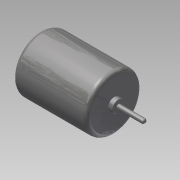
# Autodesk Inventor part: Kipas
Saved by Autodesk Inventor 2015 SP1 (Build 190203100, 203)
## iProperties
Created: 2015-02-02
Part Number: Kipas
Material: Generic
Document SubType Name: Modeling
Designer: Rafi Kurnia Putra
Density: 1 g/cm^3
Appearance: Stainless - Brushed
Mass: 17.089 g
Surface Area: 44.1561 cm^2
Volume: 17.089 cm^3
Author: Rafi Kurnia Putra
Autodesk Inventor part; units mm, degrees
ref_plane "YZ Plane" through (0, 0, 0) normal (1, 0, 0) x (0, 1, 0)
ref_plane "XZ Plane" through (0, 0, 0) normal (0, 1, 0) x (-1, 0, 0)
ref_plane "XY Plane" through (0, 0, 0) normal (0, 0, 1) x (1, 0, 0)
sketch "Sketch1" plane through (0, 0, 0) normal (0, 0, 1) x (1, 0, 0)
  circle A0 centre (0, 0) radius 12.685
  circle A1 centre (0, 0) radius 2.83
  circle A2 centre (0, 0) radius 1.05
  dimension "d0" = 25.37
  dimension "d1" = 5.66
  dimension "d2" = 2.1
  constraints: 3 centre point, 3 coincident
  measures "d0" diameter of A0
  measures "d1" diameter of A1
  measures "d2" diameter of A2
extrude "Extrusion1" add sketch "Sketch1" along normal blind 33.86 contours A0 | A1 | A2
extrude "Extrusion2" add sketch "Sketch1" against normal blind 2 contours A1
extrude "Extrusion3" add sketch "Sketch1" against normal blind 14.28 contours A2
fillet "Fillet1" radius 2 2 edges at (-12.685, 0, 0) (-12.685, 0, 33.86)
fillet "Fillet2" radius 0.25 1 edges at (-2.83, 0, -2)
fillet "Fillet3" radius 1 1 edges at (-1.05, 0, -14.28)
sketch "Sketch2" plane through (0, 0, 33.86) normal (0, 0, 1) x (1, 0, 0)
  circle A0 centre (0, 0) radius 1.05 projected
  circle A1 centre (0, 0) radius 1
  circle A2 centre (0, 0) radius 2.83
  dimension "d12" = 2
  constraints: 2 centre point, 2 coincident
  measures "d12" diameter of A1
extrude "Extrusion4" add sketch "Sketch2" along normal blind 2 contours A2
extrude "Extrusion5" add sketch "Sketch2" along normal blind 2.62 contours A1
fillet "Fillet4" radius 0.25 1 edges at (-2.83, 0, 35.86)
fillet "Fillet5" radius 1 1 edges at (-1, 0, 36.48)
sketch "Sketch4" plane through (0, 0, 33.86) normal (0, 0, 1) x (1, 0, 0)
  circle A0 centre (0, 0) radius 2.83 projected
  circle A1 centre (0, 0) radius 3.6056
  line L0 (-4.1941, 0.5305) -> (-4.1946, 0.524)
  spline S0 degree 2 poles (-4.1946, 0.524) (-4.1996, 0.5098) (-4.2034, 0.4784) (-4.2049, 0.4565) knots 0 0 0 1 2 2 2
  spline S1 degree 2 poles (-4.2049, 0.4565) (-4.2084, 0.4056) (-4.1708, 0.3023) (-4.1303, 0.254) knots 0 0 0 1 2 2 2
  line L1 (-4.1303, 0.254) -> (-3.5991, 0.2175)
  line L2 (-3.5991, 0.2175) -> (-3.6078, 0.0914)
  line L3 (-3.6078, 0.0914) -> (-4.3564, 0.1428)
  line L4 (-4.3564, 0.1428) -> (-4.3477, 0.269)
  line L5 (-4.3477, 0.269) -> (-4.2362, 0.2613)
  spline S2 degree 2 poles (-4.2362, 0.2613) (-4.2929, 0.3342) (-4.336, 0.4404) (-4.3326, 0.4889) knots 0 0 0 1 2 2 2
  spline S3 degree 2 poles (-4.3326, 0.4889) (-4.3313, 0.5083) (-4.3283, 0.5276) (-4.3251, 0.5395) knots 0 0 0 1 2 2 2
  line L6 (-4.3251, 0.5395) -> (-4.1941, 0.5305)
  spline S4 degree 2 poles (-3.5469, 1.0102) (-3.5395, 0.9926) (-3.5123, 0.9326) (-3.5062, 0.9061) knots 0 0 0 1 2 2 2
  spline S5 degree 2 poles (-3.5062, 0.9061) (-3.4967, 0.8697) (-3.4932, 0.8046) (-3.5065, 0.7495) knots 0 0 0 1 2 2 2
  spline S6 degree 2 poles (-3.5065, 0.7495) (-3.5174, 0.7046) (-3.5709, 0.6317) (-3.609, 0.6084) knots 0 0 0 1 2 2 2
  spline S7 degree 2 poles (-3.609, 0.6084) (-3.646, 0.5864) (-3.7428, 0.5723) (-3.7916, 0.5841) knots 0 0 0 1 2 2 2
  spline S8 degree 2 poles (-3.7916, 0.5841) (-3.8672, 0.6024) (-3.9589, 0.6921) (-3.9729, 0.7688) knots 0 0 0 1 2 2 2
  spline S9 degree 2 poles (-3.9729, 0.7688) (-3.9864, 0.8371) (-3.9673, 1.0093) (-3.9494, 1.1075) knots 0 0 0 1 2 2 2
  line L7 (-3.9494, 1.1075) -> (-3.9731, 1.1132)
  spline S10 degree 2 poles (-3.9731, 1.1132) (-4.0156, 1.1235) (-4.0747, 1.1102) (-4.0953, 1.0902) knots 0 0 0 1 2 2 2
  spline S11 degree 2 poles (-4.0953, 1.0902) (-4.116, 1.0702) (-4.1418, 1.0047) (-4.1506, 0.9685) knots 0 0 0 1 2 2 2
  spline S12 degree 2 poles (-4.1506, 0.9685) (-4.1609, 0.926) (-4.1635, 0.8049) (-4.1529, 0.7415) knots 0 0 0 1 2 2 2
  line L8 (-4.1529, 0.7415) -> (-4.1546, 0.7344)
  line L9 (-4.1546, 0.7344) -> (-4.2799, 0.7647)
  spline S13 degree 2 poles (-4.2799, 0.7647) (-4.2812, 0.8008) (-4.2741, 0.9333) (-4.2591, 0.9956) knots 0 0 0 1 2 2 2
  spline S14 degree 2 poles (-4.2591, 0.9956) (-4.2408, 1.0712) (-4.1923, 1.1687) (-4.1516, 1.2022) knots 0 0 0 1 2 2 2
  spline S15 degree 2 poles (-4.1516, 1.2022) (-4.112, 1.2351) (-4.0072, 1.2515) (-3.9386, 1.2349) knots 0 0 0 1 2 2 2
  line L10 (-3.9386, 1.2349) -> (-3.44, 1.1144)
  line L11 (-3.44, 1.1144) -> (-3.4697, 0.9915)
  line L12 (-3.4697, 0.9915) -> (-3.5469, 1.0102)
  line L13 (-3.6493, 1.0349) -> (-3.8518, 1.0839)
  spline S16 degree 2 poles (-3.8518, 1.0839) (-3.8585, 1.0388) (-3.8773, 0.9025) (-3.8747, 0.8577) knots 0 0 0 1 2 2 2
  spline S17 degree 2 poles (-3.8747, 0.8577) (-3.8716, 0.8052) (-3.8248, 0.7264) (-3.7696, 0.713) knots 0 0 0 1 2 2 2
  spline S18 degree 2 poles (-3.7696, 0.713) (-3.7066, 0.6978) (-3.6257, 0.7533) (-3.6093, 0.821) knots 0 0 0 1 2 2 2
  spline S19 degree 2 poles (-3.6093, 0.821) (-3.5954, 0.8785) (-3.6222, 0.985) (-3.6493, 1.0349) knots 0 0 0 1 2 2 2
  line L14 (-4.0695, 2.0028) -> (-4.072, 1.9968)
  spline S20 degree 2 poles (-4.072, 1.9968) (-4.0846, 1.9837) (-4.1198, 1.9299) (-4.1296, 1.9068) knots 0 0 0 1 2 2 2
  spline S21 degree 2 poles (-4.1296, 1.9068) (-4.1607, 1.8337) (-4.1216, 1.7432) (-4.0351, 1.7064) knots 0 0 0 1 2 2 2
  line L15 (-4.0351, 1.7064) -> (-4.012, 1.6966)
  line L16 (-4.012, 1.6966) -> (-3.9303, 1.8891)
  line L17 (-3.9303, 1.8891) -> (-3.834, 1.8482)
  line L18 (-3.834, 1.8482) -> (-3.9142, 1.6595)
  line L19 (-3.9142, 1.6595) -> (-3.3197, 1.407)
  line L20 (-3.3197, 1.407) -> (-3.3691, 1.2907)
  line L21 (-3.3691, 1.2907) -> (-3.9636, 1.5431)
  line L22 (-3.9636, 1.5431) -> (-3.9968, 1.4648)
  line L23 (-3.9968, 1.4648) -> (-4.0931, 1.5057)
  line L24 (-4.0931, 1.5057) -> (-4.0598, 1.584)
  line L25 (-4.0598, 1.584) -> (-4.0829, 1.5938)
  spline S22 degree 2 poles (-4.0829, 1.5938) (-4.2067, 1.6464) (-4.2855, 1.8216) (-4.238, 1.9335) knots 0 0 0 1 2 2 2
  spline S23 degree 2 poles (-4.238, 1.9335) (-4.2244, 1.9655) (-4.1914, 2.0246) (-4.1762, 2.0481) knots 0 0 0 1 2 2 2
  line L26 (-4.1762, 2.0481) -> (-4.0695, 2.0028)
  line L27 (-3.1163, 1.8146) -> (-3.178, 1.7043)
  line L28 (-3.178, 1.7043) -> (-3.8329, 2.0705)
  line L29 (-3.8329, 2.0705) -> (-3.7713, 2.1808)
  line L30 (-3.7713, 2.1808) -> (-3.1163, 1.8146)
  line L31 (-3.8758, 2.2495) -> (-3.9458, 2.1243)
  line L32 (-3.9458, 2.1243) -> (-4.0604, 2.1884)
  line L33 (-4.0604, 2.1884) -> (-3.9904, 2.3136)
  line L34 (-3.9904, 2.3136) -> (-3.8758, 2.2495)
  line L35 (-2.6508, 2.472) -> (-2.7511, 2.3395)
  line L36 (-2.7511, 2.3395) -> (-3.2082, 2.3359)
  line L37 (-3.2082, 2.3359) -> (-3.1997, 2.2665)
  line L38 (-3.1997, 2.2665) -> (-2.9497, 2.0772)
  line L39 (-2.9497, 2.0772) -> (-3.026, 1.9764)
  line L40 (-3.026, 1.9764) -> (-3.8588, 2.6069)
  line L41 (-3.8588, 2.6069) -> (-3.7825, 2.7077)
  line L42 (-3.7825, 2.7077) -> (-3.2953, 2.3389)
  line L43 (-3.2953, 2.3389) -> (-3.3689, 2.7666)
  line L44 (-3.3689, 2.7666) -> (-3.274, 2.892)
  line L45 (-3.274, 2.892) -> (-3.2099, 2.4572)
  line L46 (-3.2099, 2.4572) -> (-2.6508, 2.472)
  line L47 (-2.1644, 2.8983) -> (-2.2593, 2.8148)
  line L48 (-2.2593, 2.8148) -> (-2.3139, 2.8768)
  spline S24 degree 2 poles (-2.3139, 2.8768) (-2.324, 2.7999) (-2.3676, 2.6913) (-2.4162, 2.6484) knots 0 0 0 1 2 2 2
  spline S25 degree 2 poles (-2.4162, 2.6484) (-2.4527, 2.6163) (-2.5392, 2.5833) (-2.586, 2.5886) knots 0 0 0 1 2 2 2
  spline S26 degree 2 poles (-2.586, 2.5886) (-2.6333, 2.5933) (-2.7302, 2.6494) (-2.7806, 2.7065) knots 0 0 0 1 2 2 2
  line L49 (-2.7806, 2.7065) -> (-3.1025, 3.072)
  line L50 (-3.1025, 3.072) -> (-3.0077, 3.1556)
  line L51 (-3.0077, 3.1556) -> (-2.7248, 2.8345)
  spline S27 degree 2 poles (-2.7248, 2.8345) (-2.6852, 2.7895) (-2.6265, 2.7364) (-2.5957, 2.7247) knots 0 0 0 1 2 2 2
  spline S28 degree 2 poles (-2.5957, 2.7247) (-2.5649, 2.713) (-2.5077, 2.7277) (-2.4706, 2.7604) knots 0 0 0 1 2 2 2
  spline S29 degree 2 poles (-2.4706, 2.7604) (-2.4359, 2.7909) (-2.3923, 2.8996) (-2.3846, 2.9571) knots 0 0 0 1 2 2 2
  line L52 (-2.3846, 2.9571) -> (-2.7553, 3.3779)
  line L53 (-2.7553, 3.3779) -> (-2.6605, 3.4614)
  line L54 (-2.6605, 3.4614) -> (-2.1644, 2.8983)
  line L55 (-1.9912, 3.7292) -> (-1.9968, 3.7258)
  spline S30 degree 2 poles (-1.9968, 3.7258) (-2.0113, 3.7217) (-2.0391, 3.7066) (-2.0578, 3.6952) knots 0 0 0 1 2 2 2
  spline S31 degree 2 poles (-2.0578, 3.6952) (-2.1014, 3.6687) (-2.164, 3.5783) (-2.18, 3.5173) knots 0 0 0 1 2 2 2
  line L56 (-2.18, 3.5173) -> (-1.9028, 3.0627)
  line L57 (-1.9028, 3.0627) -> (-2.0107, 2.9969)
  line L58 (-2.0107, 2.9969) -> (-2.4014, 3.6376)
  line L59 (-2.4014, 3.6376) -> (-2.2935, 3.7034)
  line L60 (-2.2935, 3.7034) -> (-2.2352, 3.6079)
  spline S32 degree 2 poles (-2.2352, 3.6079) (-2.2085, 3.6964) (-2.1468, 3.7929) (-2.1053, 3.8182) knots 0 0 0 1 2 2 2
  spline S33 degree 2 poles (-2.1053, 3.8182) (-2.0887, 3.8283) (-2.0712, 3.837) (-2.0596, 3.8413) knots 0 0 0 1 2 2 2
  line L61 (-2.0596, 3.8413) -> (-1.9912, 3.7292)
  line L62 (-1.037, 3.466) -> (-1.1547, 3.4199)
  line L63 (-1.1547, 3.4199) -> (-1.3106, 3.8184)
  spline S34 degree 2 poles (-1.3106, 3.8184) (-1.3295, 3.8667) (-1.3711, 3.9461) (-1.3944, 3.9657) knots 0 0 0 1 2 2 2
  spline S35 degree 2 poles (-1.3944, 3.9657) (-1.4191, 3.9865) (-1.4805, 3.9921) (-1.5242, 3.975) knots 0 0 0 1 2 2 2
  spline S36 degree 2 poles (-1.5242, 3.975) (-1.568, 3.9578) (-1.6425, 3.8747) (-1.6723, 3.8196) knots 0 0 0 1 2 2 2
  line L64 (-1.6723, 3.8196) -> (-1.4679, 3.2974)
  line L65 (-1.4679, 3.2974) -> (-1.5856, 3.2513)
  line L66 (-1.5856, 3.2513) -> (-1.8591, 3.9501)
  line L67 (-1.8591, 3.9501) -> (-1.7414, 3.9962)
  line L68 (-1.7414, 3.9962) -> (-1.7109, 3.9184)
  spline S37 degree 2 poles (-1.7109, 3.9184) (-1.6767, 3.9867) (-1.5943, 4.0763) (-1.537, 4.0988) knots 0 0 0 1 2 2 2
  spline S38 degree 2 poles (-1.537, 4.0988) (-1.4344, 4.1389) (-1.265, 4.0486) (-1.2145, 3.9195) knots 0 0 0 1 2 2 2
  line L69 (-1.2145, 3.9195) -> (-1.037, 3.466)
  line L70 (-0.7376, 3.5299) -> (-0.8609, 3.5018)
  line L71 (-0.8609, 3.5018) -> (-1.0272, 4.2336)
  line L72 (-1.0272, 4.2336) -> (-0.9039, 4.2616)
  line L73 (-0.9039, 4.2616) -> (-0.7376, 3.5299)
  line L74 (-0.9229, 4.3853) -> (-1.0628, 4.3535)
  line L75 (-1.0628, 4.3535) -> (-1.0919, 4.4815)
  line L76 (-1.0919, 4.4815) -> (-0.952, 4.5133)
  line L77 (-0.952, 4.5133) -> (-0.9229, 4.3853)
  spline S39 degree 2 poles (-0.1468, 3.685) (-0.1613, 3.6725) (-0.2097, 3.628) (-0.233, 3.6139) knots 0 0 0 1 2 2 2
  spline S40 degree 2 poles (-0.233, 3.6139) (-0.2647, 3.5935) (-0.3254, 3.5699) (-0.3819, 3.5653) knots 0 0 0 1 2 2 2
  spline S41 degree 2 poles (-0.3819, 3.5653) (-0.428, 3.5617) (-0.514, 3.5897) (-0.548, 3.6187) knots 0 0 0 1 2 2 2
  spline S42 degree 2 poles (-0.548, 3.6187) (-0.5803, 3.647) (-0.624, 3.7345) (-0.628, 3.7846) knots 0 0 0 1 2 2 2
  spline S43 degree 2 poles (-0.628, 3.7846) (-0.6342, 3.8621) (-0.5776, 3.9773) (-0.5091, 4.0145) knots 0 0 0 1 2 2 2
  spline S44 degree 2 poles (-0.5091, 4.0145) (-0.4484, 4.0486) (-0.2789, 4.0842) (-0.18, 4.0978) knots 0 0 0 1 2 2 2
  line L78 (-0.18, 4.0978) -> (-0.1819, 4.122)
  spline S45 degree 2 poles (-0.1819, 4.122) (-0.1854, 4.1657) (-0.2164, 4.2176) (-0.2419, 4.231) knots 0 0 0 1 2 2 2
  spline S46 degree 2 poles (-0.2419, 4.231) (-0.2674, 4.2444) (-0.3376, 4.2486) (-0.3748, 4.2456) knots 0 0 0 1 2 2 2
  spline S47 degree 2 poles (-0.3748, 4.2456) (-0.4184, 4.2421) (-0.5343, 4.2068) (-0.5912, 4.177) knots 0 0 0 1 2 2 2
  line L79 (-0.5912, 4.177) -> (-0.5985, 4.1764)
  line L80 (-0.5985, 4.1764) -> (-0.6088, 4.3048)
  spline S48 degree 2 poles (-0.6088, 4.3048) (-0.5748, 4.3173) (-0.4467, 4.352) (-0.3829, 4.3571) knots 0 0 0 1 2 2 2
  spline S49 degree 2 poles (-0.3829, 4.3571) (-0.3054, 4.3633) (-0.1976, 4.3476) (-0.1531, 4.3195) knots 0 0 0 1 2 2 2
  spline S50 degree 2 poles (-0.1531, 4.3195) (-0.1094, 4.2921) (-0.0612, 4.1976) (-0.0555, 4.1273) knots 0 0 0 1 2 2 2
  line L81 (-0.0555, 4.1273) -> (-0.0145, 3.616)
  line L82 (-0.0145, 3.616) -> (-0.1405, 3.6059)
  line L83 (-0.1405, 3.6059) -> (-0.1468, 3.685)
  line L84 (-0.1553, 3.7901) -> (-0.1719, 3.9977)
  spline S51 degree 2 poles (-0.1719, 3.9977) (-0.2168, 3.99) (-0.3523, 3.9653) (-0.394, 3.9489) knots 0 0 0 1 2 2 2
  spline S52 degree 2 poles (-0.394, 3.9489) (-0.4429, 3.9295) (-0.5032, 3.8605) (-0.4986, 3.8039) knots 0 0 0 1 2 2 2
  spline S53 degree 2 poles (-0.4986, 3.8039) (-0.4935, 3.7393) (-0.4155, 3.6797) (-0.346, 3.6853) knots 0 0 0 1 2 2 2
  spline S54 degree 2 poles (-0.346, 3.6853) (-0.2871, 3.69) (-0.1942, 3.7487) (-0.1553, 3.7901) knots 0 0 0 1 2 2 2
  point P0 (0, 3.6056)
  point P1 (-3.6056, 0)
  constraints: 2 point on circle, 1 centre point, 1 other
extrude "Extrusion6" cut sketch "Sketch4" against normal blind 10 contours L2 L3 L4 L5 S2 S3 L6 L0 S0 S1 L1 | L20 L21 L22 L23 L24 L25 S22 S23 L26 L14 S20 S21 L15 L16 L17 L18 L19 | L57 L58 L59 L60 S32 S33 L61 L55 S30 S31 L56 | A1 L71 L72 L73 | S41 S42 S43 S44 L78 S45 S46 S47 L79 L80 S48 S49 S50 L81 L82 L83 S39 S40 A1 | A1 S40 S41 | S24 S25 A1 | A1 S25 S26 L49 L50 L51 S27 S28 S29 L52 L53 L54 L47 L48 S24 | A1 L28 L29 L30 | S6 S7 S8 S9 L7 S10 S11 S12 L8 L9 S13 S14 S15 L10 L11 L12 S4 S5 A1 | A1 S5 S6 | L31 L32 L33 L34 | L35 L36 L37 L38 L39 L40 L41 L42 L43 L44 L45 L46 | L62 L63 S34 S35 S36 L64 L65 L66 L67 L68 S37 S38 L69 | L74 L75 L76 L77
sketch "Sketch5" plane through (0, 0, 0) normal (0, 0, -1) x (-1, 0, 0)
  circle A0 centre (0, 0) radius 10.685 projected
  line L0 (-4.7473, -8.884) -> (-4.7529, -8.8808)
  spline S0 degree 2 poles (-4.7529, -8.8808) (-4.7636, -8.8701) (-4.7903, -8.8531) (-4.8094, -8.8424) knots 0 0 0 1 2 2 2
  spline S1 degree 2 poles (-4.8094, -8.8424) (-4.8538, -8.8172) (-4.9632, -8.8065) (-5.0242, -8.8223) knots 0 0 0 1 2 2 2
  line L1 (-5.0242, -8.8223) -> (-5.2864, -9.2857)
  line L2 (-5.2864, -9.2857) -> (-5.3964, -9.2235)
  line L3 (-5.3964, -9.2235) -> (-5.027, -8.5703)
  line L4 (-5.027, -8.5703) -> (-4.9169, -8.6325)
  line L5 (-4.9169, -8.6325) -> (-4.972, -8.7299)
  spline S2 degree 2 poles (-4.972, -8.7299) (-4.8817, -8.7102) (-4.7674, -8.7171) (-4.7251, -8.7411) knots 0 0 0 1 2 2 2
  spline S3 degree 2 poles (-4.7251, -8.7411) (-4.7081, -8.7506) (-4.692, -8.7616) (-4.6826, -8.7697) knots 0 0 0 1 2 2 2
  line L6 (-4.6826, -8.7697) -> (-4.7473, -8.884)
  spline S4 degree 2 poles (-4.5536, -9.5794) (-4.5724, -9.5828) (-4.6368, -9.5962) (-4.664, -9.5964) knots 0 0 0 1 2 2 2
  spline S5 degree 2 poles (-4.664, -9.5964) (-4.7017, -9.5977) (-4.7659, -9.5868) (-4.8168, -9.5618) knots 0 0 0 1 2 2 2
  spline S6 degree 2 poles (-4.8168, -9.5618) (-4.8582, -9.5414) (-4.9177, -9.4732) (-4.9321, -9.4309) knots 0 0 0 1 2 2 2
  spline S7 degree 2 poles (-4.9321, -9.4309) (-4.9454, -9.39) (-4.938, -9.2925) (-4.9158, -9.2474) knots 0 0 0 1 2 2 2
  spline S8 degree 2 poles (-4.9158, -9.2474) (-4.8814, -9.1776) (-4.7738, -9.1078) (-4.6959, -9.1109) knots 0 0 0 1 2 2 2
  spline S9 degree 2 poles (-4.6959, -9.1109) (-4.6263, -9.1127) (-4.4625, -9.169) (-4.3706, -9.208) knots 0 0 0 1 2 2 2
  line L7 (-4.3706, -9.208) -> (-4.3598, -9.1861)
  spline S10 degree 2 poles (-4.3598, -9.1861) (-4.3405, -9.1469) (-4.3405, -9.0864) (-4.3555, -9.0618) knots 0 0 0 1 2 2 2
  spline S11 degree 2 poles (-4.3555, -9.0618) (-4.3705, -9.0373) (-4.4287, -8.9977) (-4.4622, -8.9813) knots 0 0 0 1 2 2 2
  spline S12 degree 2 poles (-4.4622, -8.9813) (-4.5014, -8.9619) (-4.619, -8.9329) (-4.6832, -8.9293) knots 0 0 0 1 2 2 2
  line L8 (-4.6832, -8.9293) -> (-4.6897, -8.9261)
  line L9 (-4.6897, -8.9261) -> (-4.6328, -8.8105)
  spline S13 degree 2 poles (-4.6328, -8.8105) (-4.5972, -8.8172) (-4.4694, -8.853) (-4.412, -8.8813) knots 0 0 0 1 2 2 2
  spline S14 degree 2 poles (-4.412, -8.8813) (-4.3422, -8.9157) (-4.2577, -8.9844) (-4.2339, -9.0314) knots 0 0 0 1 2 2 2
  spline S15 degree 2 poles (-4.2339, -9.0314) (-4.2104, -9.0773) (-4.2174, -9.1831) (-4.2486, -9.2464) knots 0 0 0 1 2 2 2
  line L10 (-4.2486, -9.2464) -> (-4.4753, -9.7065)
  line L11 (-4.4753, -9.7065) -> (-4.5887, -9.6507)
  line L12 (-4.5887, -9.6507) -> (-4.5536, -9.5794)
  line L13 (-4.507, -9.4849) -> (-4.415, -9.2981)
  spline S16 degree 2 poles (-4.415, -9.2981) (-4.4575, -9.2817) (-4.5864, -9.2335) (-4.6307, -9.2262) knots 0 0 0 1 2 2 2
  spline S17 degree 2 poles (-4.6307, -9.2262) (-4.6826, -9.2178) (-4.7697, -9.2462) (-4.7948, -9.2971) knots 0 0 0 1 2 2 2
  spline S18 degree 2 poles (-4.7948, -9.2971) (-4.8235, -9.3552) (-4.787, -9.4463) (-4.7245, -9.4771) knots 0 0 0 1 2 2 2
  spline S19 degree 2 poles (-4.7245, -9.4771) (-4.6715, -9.5033) (-4.5617, -9.5005) (-4.507, -9.4849) knots 0 0 0 1 2 2 2
  line L14 (-3.5881, -9.0822) -> (-3.594, -9.0796)
  spline S20 degree 2 poles (-3.594, -9.0796) (-3.6072, -9.067) (-3.6609, -9.0318) (-3.684, -9.022) knots 0 0 0 1 2 2 2
  spline S21 degree 2 poles (-3.684, -9.022) (-3.7571, -8.9909) (-3.8476, -9.0299) (-3.8844, -9.1164) knots 0 0 0 1 2 2 2
  line L15 (-3.8844, -9.1164) -> (-3.8943, -9.1395)
  line L16 (-3.8943, -9.1395) -> (-3.7019, -9.2214)
  line L17 (-3.7019, -9.2214) -> (-3.7428, -9.3176)
  line L18 (-3.7428, -9.3176) -> (-3.9315, -9.2373)
  line L19 (-3.9315, -9.2373) -> (-4.1842, -9.8317)
  line L20 (-4.1842, -9.8317) -> (-4.3006, -9.7822)
  line L21 (-4.3006, -9.7822) -> (-4.0478, -9.1878)
  line L22 (-4.0478, -9.1878) -> (-4.1261, -9.1545)
  line L23 (-4.1261, -9.1545) -> (-4.0852, -9.0583)
  line L24 (-4.0852, -9.0583) -> (-4.0069, -9.0916)
  line L25 (-4.0069, -9.0916) -> (-3.997, -9.0685)
  spline S22 degree 2 poles (-3.997, -9.0685) (-3.9444, -8.9447) (-3.7691, -8.866) (-3.6573, -8.9136) knots 0 0 0 1 2 2 2
  spline S23 degree 2 poles (-3.6573, -8.9136) (-3.6252, -8.9272) (-3.5662, -8.9603) (-3.5427, -8.9755) knots 0 0 0 1 2 2 2
  line L26 (-3.5427, -8.9755) -> (-3.5881, -9.0822)
  line L27 (-3.7609, -10.0015) -> (-3.8789, -9.9563)
  line L28 (-3.8789, -9.9563) -> (-3.6107, -9.2555)
  line L29 (-3.6107, -9.2555) -> (-3.4926, -9.3006)
  line L30 (-3.4926, -9.3006) -> (-3.7609, -10.0015)
  line L31 (-3.4396, -9.1873) -> (-3.5736, -9.136)
  line L32 (-3.5736, -9.136) -> (-3.5267, -9.0134)
  line L33 (-3.5267, -9.0134) -> (-3.3927, -9.0647)
  line L34 (-3.3927, -9.0647) -> (-3.4396, -9.1873)
  line L35 (-2.9974, -10.2627) -> (-3.1551, -10.2106)
  line L36 (-3.1551, -10.2106) -> (-3.3063, -9.7792)
  line L37 (-3.3063, -9.7792) -> (-3.3692, -9.8097)
  line L38 (-3.3692, -9.8097) -> (-3.4676, -10.1075)
  line L39 (-3.4676, -10.1075) -> (-3.5876, -10.0678)
  line L40 (-3.5876, -10.0678) -> (-3.2602, -9.0759)
  line L41 (-3.2602, -9.0759) -> (-3.1401, -9.1155)
  line L42 (-3.1401, -9.1155) -> (-3.3316, -9.6958)
  line L43 (-3.3316, -9.6958) -> (-2.9507, -9.4879)
  line L44 (-2.9507, -9.4879) -> (-2.8014, -9.5371)
  line L45 (-2.8014, -9.5371) -> (-3.1921, -9.7384)
  line L46 (-3.1921, -9.7384) -> (-2.9974, -10.2627)
  line L47 (-2.3708, -10.4227) -> (-2.4933, -10.3914)
  line L48 (-2.4933, -10.3914) -> (-2.4727, -10.3113)
  spline S24 degree 2 poles (-2.4727, -10.3113) (-2.5419, -10.3462) (-2.6563, -10.3713) (-2.7191, -10.3552) knots 0 0 0 1 2 2 2
  spline S25 degree 2 poles (-2.7191, -10.3552) (-2.7662, -10.3431) (-2.8421, -10.2902) (-2.8641, -10.2486) knots 0 0 0 1 2 2 2
  spline S26 degree 2 poles (-2.8641, -10.2486) (-2.8868, -10.2068) (-2.895, -10.0951) (-2.8761, -10.0213) knots 0 0 0 1 2 2 2
  line L49 (-2.8761, -10.0213) -> (-2.7551, -9.5495)
  line L50 (-2.7551, -9.5495) -> (-2.6327, -9.5809)
  line L51 (-2.6327, -9.5809) -> (-2.7389, -9.9954)
  spline S27 degree 2 poles (-2.7389, -9.9954) (-2.7538, -10.0535) (-2.7647, -10.1319) (-2.757, -10.1639) knots 0 0 0 1 2 2 2
  spline S28 degree 2 poles (-2.757, -10.1639) (-2.7494, -10.196) (-2.705, -10.235) (-2.6571, -10.2473) knots 0 0 0 1 2 2 2
  spline S29 degree 2 poles (-2.6571, -10.2473) (-2.6124, -10.2588) (-2.498, -10.2337) (-2.4462, -10.2077) knots 0 0 0 1 2 2 2
  line L52 (-2.4462, -10.2077) -> (-2.3069, -9.6645)
  line L53 (-2.3069, -9.6645) -> (-2.1845, -9.6958)
  line L54 (-2.1845, -9.6958) -> (-2.3708, -10.4227)
  line L55 (-1.6835, -9.9311) -> (-1.6898, -9.9299)
  spline S30 degree 2 poles (-1.6898, -9.9299) (-1.7034, -9.9232) (-1.7341, -9.9155) (-1.7556, -9.9114) knots 0 0 0 1 2 2 2
  spline S31 degree 2 poles (-1.7556, -9.9114) (-1.8057, -9.9016) (-1.9128, -9.9262) (-1.9657, -9.9605) knots 0 0 0 1 2 2 2
  line L56 (-1.9657, -9.9605) -> (-2.0673, -10.4832)
  line L57 (-2.0673, -10.4832) -> (-2.1914, -10.459)
  line L58 (-2.1914, -10.459) -> (-2.0482, -9.7224)
  line L59 (-2.0482, -9.7224) -> (-1.9241, -9.7465)
  line L60 (-1.9241, -9.7465) -> (-1.9455, -9.8563)
  spline S32 degree 2 poles (-1.9455, -9.8563) (-1.8661, -9.809) (-1.7555, -9.7793) (-1.7078, -9.7886) knots 0 0 0 1 2 2 2
  spline S33 degree 2 poles (-1.7078, -9.7886) (-1.6887, -9.7923) (-1.6699, -9.7976) (-1.6584, -9.8023) knots 0 0 0 1 2 2 2
  line L61 (-1.6584, -9.8023) -> (-1.6835, -9.9311)
  line L62 (-1.1204, -10.6303) -> (-1.2457, -10.6135)
  line L63 (-1.2457, -10.6135) -> (-1.189, -10.1894)
  spline S34 degree 2 poles (-1.189, -10.1894) (-1.1821, -10.138) (-1.18, -10.0484) (-1.1909, -10.0199) knots 0 0 0 1 2 2 2
  spline S35 degree 2 poles (-1.1909, -10.0199) (-1.2024, -9.9898) (-1.2533, -9.9552) (-1.2999, -9.9489) knots 0 0 0 1 2 2 2
  spline S36 degree 2 poles (-1.2999, -9.9489) (-1.3465, -9.9427) (-1.452, -9.9793) (-1.5047, -10.0131) knots 0 0 0 1 2 2 2
  line L64 (-1.5047, -10.0131) -> (-1.579, -10.569)
  line L65 (-1.579, -10.569) -> (-1.7043, -10.5522)
  line L66 (-1.7043, -10.5522) -> (-1.6049, -9.8084)
  line L67 (-1.6049, -9.8084) -> (-1.4796, -9.8252)
  line L68 (-1.4796, -9.8252) -> (-1.4907, -9.9079)
  spline S37 degree 2 poles (-1.4907, -9.9079) (-1.4277, -9.8648) (-1.3122, -9.8263) (-1.2511, -9.8345) knots 0 0 0 1 2 2 2
  spline S38 degree 2 poles (-1.2511, -9.8345) (-1.1419, -9.8491) (-1.0375, -10.0102) (-1.0559, -10.1475) knots 0 0 0 1 2 2 2
  line L69 (-1.0559, -10.1475) -> (-1.1204, -10.6303)
  line L70 (-0.815, -10.6541) -> (-0.941, -10.6437)
  line L71 (-0.941, -10.6437) -> (-0.8793, -9.8958)
  line L72 (-0.8793, -9.8958) -> (-0.7533, -9.9062)
  line L73 (-0.7533, -9.9062) -> (-0.815, -10.6541)
  line L74 (-0.7342, -9.7826) -> (-0.8771, -9.7708)
  line L75 (-0.8771, -9.7708) -> (-0.8663, -9.6399)
  line L76 (-0.8663, -9.6399) -> (-0.7234, -9.6517)
  line L77 (-0.7234, -9.6517) -> (-0.7342, -9.7826)
  spline S39 degree 2 poles (-0.2095, -10.6046) (-0.2253, -10.6154) (-0.2785, -10.6541) (-0.3032, -10.6654) knots 0 0 0 1 2 2 2
  spline S40 degree 2 poles (-0.3032, -10.6654) (-0.337, -10.6821) (-0.4, -10.6987) (-0.4567, -10.6967) knots 0 0 0 1 2 2 2
  spline S41 degree 2 poles (-0.4567, -10.6967) (-0.5029, -10.6952) (-0.5851, -10.6575) (-0.6156, -10.6249) knots 0 0 0 1 2 2 2
  spline S42 degree 2 poles (-0.6156, -10.6249) (-0.6445, -10.5931) (-0.6779, -10.5012) (-0.6762, -10.4509) knots 0 0 0 1 2 2 2
  spline S43 degree 2 poles (-0.6762, -10.4509) (-0.6736, -10.3732) (-0.6043, -10.2653) (-0.5319, -10.2361) knots 0 0 0 1 2 2 2
  spline S44 degree 2 poles (-0.5319, -10.2361) (-0.4678, -10.2091) (-0.2953, -10.193) (-0.1955, -10.1907) knots 0 0 0 1 2 2 2
  line L78 (-0.1955, -10.1907) -> (-0.1947, -10.1664)
  spline S45 degree 2 poles (-0.1947, -10.1664) (-0.1932, -10.1227) (-0.2181, -10.0675) (-0.2419, -10.0513) knots 0 0 0 1 2 2 2
  spline S46 degree 2 poles (-0.2419, -10.0513) (-0.2657, -10.0351) (-0.335, -10.023) (-0.3723, -10.0217) knots 0 0 0 1 2 2 2
  spline S47 degree 2 poles (-0.3723, -10.0217) (-0.416, -10.0203) (-0.5351, -10.0422) (-0.5951, -10.0653) knots 0 0 0 1 2 2 2
  line L79 (-0.5951, -10.0653) -> (-0.6024, -10.0651)
  line L80 (-0.6024, -10.0651) -> (-0.598, -9.9363)
  spline S48 degree 2 poles (-0.598, -9.9363) (-0.5629, -9.9277) (-0.4317, -9.9078) (-0.3677, -9.91) knots 0 0 0 1 2 2 2
  spline S49 degree 2 poles (-0.3677, -9.91) (-0.2899, -9.9126) (-0.1846, -9.9405) (-0.1436, -9.9735) knots 0 0 0 1 2 2 2
  spline S50 degree 2 poles (-0.1436, -9.9735) (-0.1033, -10.0057) (-0.0661, -10.1051) (-0.0685, -10.1755) knots 0 0 0 1 2 2 2
  line L81 (-0.0685, -10.1755) -> (-0.0859, -10.6882)
  line L82 (-0.0859, -10.6882) -> (-0.2122, -10.6839)
  line L83 (-0.2122, -10.6839) -> (-0.2095, -10.6046)
  line L84 (-0.206, -10.4993) -> (-0.1989, -10.2911)
  spline S51 degree 2 poles (-0.1989, -10.2911) (-0.2444, -10.2936) (-0.3818, -10.3028) (-0.4251, -10.3143) knots 0 0 0 1 2 2 2
  spline S52 degree 2 poles (-0.4251, -10.3143) (-0.4759, -10.328) (-0.5436, -10.3897) (-0.5455, -10.4464) knots 0 0 0 1 2 2 2
  spline S53 degree 2 poles (-0.5455, -10.4464) (-0.5477, -10.5112) (-0.477, -10.5793) (-0.4074, -10.5817) knots 0 0 0 1 2 2 2
  spline S54 degree 2 poles (-0.4074, -10.5817) (-0.3483, -10.5837) (-0.2494, -10.5359) (-0.206, -10.4993) knots 0 0 0 1 2 2 2
  constraints: 1 other
extrude "Extrusion7" cut sketch "Sketch5" against normal blind 10 contours L3 L4 L5 S2 S3 L6 L0 S0 S1 L1 A0 | L81 L82 A0 | A0 L83 S39 S40 S41 S42 S43 S44 L78 S45 S46 S47 L79 L80 S48 S49 S50 L81 | S6 S7 S8 S9 L7 S10 S11 S12 L8 L9 S13 S14 S15 L10 A0 L12 S4 S5 | A0 S5 S6 | S40 S41 A0 | A0 L10 L11 | A0 L71 L72 L73 | L21 L22 L23 L24 L25 S22 S23 L26 L14 S20 S21 L15 L16 L17 L18 L19 A0 | L69 L62 A0 | A0 L63 S34 S35 S36 L64 L66 L67 L68 S37 S38 L69 | L28 L29 L30 A0 | L65 L66 A0 | L40 L41 L42 L43 L44 L45 L46 A0 L36 L37 L38 | A0 L39 L40 | A0 L58 L59 L60 S32 S33 L61 L55 S30 S31 L56 | A0 L46 L35 | L54 L47 A0 | A0 L48 S24 S25 S26 L49 L50 L51 S27 S28 S29 L52 L53 L54 | A0 S24 S25 | L31 L32 L33 L34 | L74 L75 L76 L77
sketch "Sketch6" plane through (0, 0, 0) normal (0, 1, 0) x (-1, 0, 0)
  line L0 (0.05, -14.28) -> (-0.05, -14.28) projected
  line L1 (0, -14.28) -> (0, -214.28)
  point P0 (0, 0)
  constraints: 2 end point, 1 midpoint, 1 vertical
body "Solid1"
